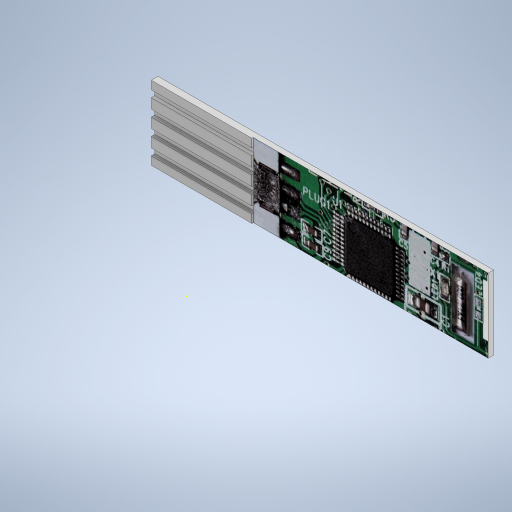
# Autodesk Inventor part: Pen2
Saved by Autodesk Inventor 2024.2 (Build 282272000, 272)
## iProperties
Created: 2024-04-15
Part Number: Pen2
Material: Acetal Resin, White
Document SubType Name: Modeling
Designer: 082220022
Density: 1.425 g/cm^3
Appearance: Default
Author: 082220022
Autodesk Inventor part; units mm, degrees
ref_plane "YZ Plane" through (0, 0, 0) normal (1, 0, 0) x (0, 1, 0)
ref_plane "XZ Plane" through (0, 0, 0) normal (0, 1, 0) x (-1, 0, 0)
ref_plane "XY Plane" through (0, 0, 0) normal (0, 0, 1) x (1, 0, 0)
sketch "Sketch1" plane through (0, 0, 0) normal (0, 0, 1) x (1, 0, 0)
  line L0 (-25, -5.5) -> (25, -5.5)
  line L1 (25, -5.5) -> (25, 5.5)
  line L2 (25, 5.5) -> (-25, 5.5)
  line L3 (-25, 5.5) -> (-25, -5.5)
  line L4 (-25, -5.5) -> (25, 5.5) construction
  line L5 (25, -5.5) -> (-25, 5.5) construction
  point P0 (0, 0)
  dimension "d0" = 50
  dimension "d1" = 11
  constraints: 12 end point, 2 midpoint, 2 parallel, 1 horizontal, 1 perpendicular
  measures "d0" distance of L2.end L1.end
  measures "d1" distance of L1.end L0.end
extrude "Extrusion1" add sketch "Sketch1" along normal mid plane 0.8
sketch "Sketch2" plane through (0, 0, 0.4) normal (0, 0, 1) x (1, 0, 0)
  line L0 (25, 5.5) -> (-25, 5.5) projected
  line L1 (-25, -5.5) -> (25, -5.5) projected
  line L2 (-25, 5.5) -> (-10, 5.5)
  line L3 (-10, 5.5) -> (-10, -5.5)
  line L4 (-10, -5.5) -> (-25, -5.5)
  line L5 (-25, -5.5) -> (-25, 5.5)
  point P0 (0, 0)
  dimension "d4" = 15
  dimension "d5" = 11
  constraints: 8 end point, 2 parallel, 1 horizontal, 1 perpendicular, 1 point on line
  measures "d4" distance of L3.end L4.end
  measures "d5" distance of L2.end L3.end
extrude "Extrusion2" add sketch "Sketch2" along normal blind 0.2
sketch "Sketch3" plane through (0, 0, 0.6) normal (0, 0, 1) x (1, 0, 0)
  line L0 (-25, 4.25) -> (-10, 4.25)
  line L1 (-10, 4.25) -> (-10, 3.25)
  line L2 (-10, 3.25) -> (-25, 3.25)
  line L3 (-25, 3.25) -> (-25, 4.25)
  line L4 (-25, 5.5) -> (-25, -5.5) projected
  line L5 (-10, 5.5) -> (-25, 5.5) projected
  line L6 (-10, 0.75) -> (-25, 0.75)
  line L7 (-10, 1.75) -> (-10, 0.75)
  line L8 (-25, 1.75) -> (-10, 1.75)
  line L9 (-25, 0.75) -> (-25, 1.75)
  line L10 (-10, -1.75) -> (-25, -1.75)
  line L11 (-10, -0.75) -> (-10, -1.75)
  line L12 (-25, -0.75) -> (-10, -0.75)
  line L13 (-25, -1.75) -> (-25, -0.75)
  line L14 (-10, -4.25) -> (-25, -4.25)
  line L15 (-10, -3.25) -> (-10, -4.25)
  line L16 (-25, -3.25) -> (-10, -3.25)
  line L17 (-25, -4.25) -> (-25, -3.25)
  point P0 (0, 0)
  dimension "d8" = 15
  dimension "d9" = 1
  dimension "d10" = 1.25
  dimension "d13" = 2.5
  constraints: 32 end point, 2 parallel, 1 collinear, 1 horizontal, 1 perpendicular, 1 vertical, 24 other
  measures "d8" distance of L1.end L2.end
  measures "d9" distance of L0.end L1.end
  measures "d10" distance between parallel lines of L0 L5
  measures "d13" distance of L1.end L6.start
extrude "Extrusion3" cut sketch "Sketch3" against normal blind 0.5
ref_plane "Work Plane1" through (0, 0, 20.4) normal (0, 0, 1) x (1, 0, 0)
sketch "Sketch4" plane through (0, 0, 20.4) normal (0, 0, 1) x (1, 0, 0)
  line L0 (-10, 5.5) -> (-25, 5.5) projected
  line L1 (-9.9335, 7.1739) -> (25.0665, 7.1739) construction
  line L2 (25.0665, 7.1739) -> (25.0665, -7.4481) construction
  line L3 (25.0665, -7.4481) -> (-9.9335, -7.4481) construction
  line L4 (-9.9335, -7.4481) -> (-9.9335, 7.1739) construction
  point P0 (0, 0)
  dimension "d56" = 35
  constraints: 2 other
  measures "d56" distance of L2.end L3.end
decal "Decal1"
sketch "Sketch5" plane through (0, 0, 20.4) normal (0, 0, 1) x (1, 0, 0)
  point P0 (0, 0)
body "Solid1"
